Autodesk Fusion 360 part; units mm, degrees
(part 5 of 21)
  spline S66 degree 5 poles (-12.249, -28.4774) (-12.2425, -28.4716) (-12.2296, -28.4599) (-12.2103, -28.4423) (-12.1846, -28.4188) (-12.1527, -28.3894) (-12.1208, -28.3599) (-12.0891, -28.3303) (-12.0576, -28.3006) (-12.0261, -28.2709) (-11.9948, -28.241) (-11.9637, -28.2111) (-11.9326, -28.1811) (-11.9018, -28.151) (-11.871, -28.1208) (-11.8404, -28.0906) (-11.8099, -28.0602) (-11.7796, -28.0298) (-11.7494, -27.9993) (-11.7194, -27.9687) (-11.6895, -27.938) (-11.6597, -27.9072) (-11.6301, -27.8763) (-11.6007, -27.8454) (-11.5714, -27.8143) (-11.5422, -27.7832) (-11.5132, -27.752) (-11.4844, -27.7207) (-11.4557, -27.6893) (-11.4272, -27.6578) (-11.3988, -27.6262) (-11.3706, -27.5946) (-11.3426, -27.5628) (-11.3147, -27.5309) (-11.287, -27.499) (-11.2595, -27.467) (-11.2321, -27.4348) (-11.2049, -27.4026) (-11.1779, -27.3703) (-11.1511, -27.3379) (-11.1244, -27.3054) (-11.098, -27.2728) (-11.0717, -27.2401) (-11.0456, -27.2073) (-11.0197, -27.1743) (-10.994, -27.1413) (-10.9685, -27.1082) (-10.9432, -27.075) (-10.9181, -27.0417) (-10.8932, -27.0083) (-10.8686, -26.9747) (-10.8441, -26.9411) (-10.8199, -26.9073) (-10.7959, -26.8735) (-10.7721, -26.8395) (-10.752, -26.8103) (-10.7367, -26.7878) (-10.7261, -26.7721) (-10.7202, -26.7633) (-10.7188, -26.7613) knots -1 -1 -1 -1 -1 -1 -0.985714 -0.971429 -0.957143 -0.942857 -0.928571 -0.914286 -0.9 -0.885714 -0.871429 -0.857143 -0.842857 -0.828571 -0.814286 -0.8 -0.785714 -0.771429 -0.757143 -0.742857 -0.728571 -0.714286 -0.7 -0.685714 -0.671429 -0.657143 -0.642857 -0.628571 -0.614286 -0.6 -0.585714 -0.571429 -0.557143 -0.542857 -0.528571 -0.514286 -0.5 -0.485714 -0.471429 -0.457143 -0.442857 -0.428571 -0.414286 -0.4 -0.385714 -0.371429 -0.357143 -0.342857 -0.328571 -0.314286 -0.3 -0.285714 -0.271429 -0.257143 -0.242857 -0.228571 -0.224488 -0.224488 -0.224488 -0.224488 -0.224488 -0.224488
  spline S67 degree 3 poles (-10.599, -26.7241) (-10.6111, -26.7193) (-10.624, -26.7169) (-10.65, -26.7172) (-10.6629, -26.7199) (-10.6838, -26.7288) (-10.6921, -26.7338) (-10.7069, -26.7461) (-10.7135, -26.7533) (-10.7188, -26.7613) knots 0 0 0 0 0.003906 0.003906 0.007813 0.007813 0.010709 0.010709 0.013605 0.013605 0.013605 0.013605
  arc A64 (-10.599, -26.7241) -> (-10.0054, -26.952) centre (0, 0) ccw
  spline S68 degree 3 poles (-9.9412, -27.0598) (-9.9393, -27.047) (-9.94, -27.0338) (-9.9464, -27.0086) (-9.952, -26.9967) (-9.9655, -26.9785) (-9.9724, -26.9716) (-9.9878, -26.96) (-9.9963, -26.9553) (-10.0054, -26.952) knots 0 0 0 0 0.003906 0.003906 0.007813 0.007813 0.010709 0.010709 0.013605 0.013605 0.013605 0.013605
  spline S69 degree 5 poles (-9.9412, -27.0598) (-9.9415, -27.0622) (-9.943, -27.0727) (-9.9456, -27.0914) (-9.9493, -27.1184) (-9.9539, -27.1536) (-9.9589, -27.1948) (-9.9638, -27.236) (-9.9683, -27.2773) (-9.9727, -27.3186) (-9.9768, -27.3601) (-9.9807, -27.4015) (-9.9843, -27.4431) (-9.9878, -27.4847) (-9.991, -27.5264) (-9.994, -27.5681) (-9.9967, -27.6099) (-9.9993, -27.6517) (-10.0016, -27.6936) (-10.0038, -27.7355) (-10.0057, -27.7775) (-10.0075, -27.8196) (-10.0091, -27.8617) (-10.0104, -27.9038) (-10.0116, -27.946) (-10.0126, -27.9882) (-10.0133, -28.0305) (-10.0139, -28.0728) (-10.0144, -28.1152) (-10.0146, -28.1576) (-10.0146, -28.2) (-10.0145, -28.2425) (-10.0142, -28.285) (-10.0137, -28.3276) (-10.0131, -28.3702) (-10.0122, -28.4128) (-10.0112, -28.4555) (-10.01, -28.4982) (-10.0087, -28.541) (-10.0072, -28.5837) (-10.0055, -28.6265) (-10.0037, -28.6694) (-10.0016, -28.7123) (-9.9995, -28.7552) (-9.9971, -28.7981) (-9.9946, -28.8411) (-9.992, -28.8841) (-9.9892, -28.9271) (-9.9862, -28.9702) (-9.983, -29.0133) (-9.9798, -29.0564) (-9.9763, -29.0996) (-9.9727, -29.1427) (-9.9689, -29.1859) (-9.965, -29.2292) (-9.961, -29.2724) (-9.9576, -29.307) (-9.955, -29.333) (-9.9532, -29.3503) (-9.9524, -29.359) knots 0.224488 0.224488 0.224488 0.224488 0.224488 0.224488 0.228571 0.242857 0.257143 0.271429 0.285714 0.3 0.314286 0.328571 0.342857 0.357143 0.371429 0.385714 0.4 0.414286 0.428571 0.442857 0.457143 0.471429 0.485714 0.5 0.514286 0.528571 0.542857 0.557143 0.571429 0.585714 0.6 0.614286 0.628571 0.642857 0.657143 0.671429 0.685714 0.7 0.714286 0.728571 0.742857 0.757143 0.771429 0.785714 0.8 0.814286 0.828571 0.842857 0.857143 0.871429 0.885714 0.9 0.914286 0.928571 0.942857 0.957143 0.971429 0.985714 1 1 1 1 1 1
  arc A65 (-9.9524, -29.359) -> (-9.2052, -29.6018) centre (0, 0) ccw
  spline S70 degree 5 poles (-9.2052, -29.6018) (-9.1994, -29.5953) (-9.1877, -29.5823) (-9.1704, -29.5628) (-9.1473, -29.5368) (-9.1186, -29.5042) (-9.09, -29.4715) (-9.0616, -29.4388) (-9.0333, -29.406) (-9.0051, -29.3731) (-8.9771, -29.3401) (-8.9493, -29.3071) (-8.9215, -29.274) (-8.894, -29.2409) (-8.8665, -29.2076) (-8.8393, -29.1743) (-8.8121, -29.141) (-8.7851, -29.1075) (-8.7583, -29.074) (-8.7316, -29.0405) (-8.7051, -29.0068) (-8.6787, -28.9731) (-8.6525, -28.9393) (-8.6265, -28.9054) (-8.6006, -28.8715) (-8.5748, -28.8375) (-8.5493, -28.8034) (-8.5239, -28.7693) (-8.4986, -28.735) (-8.4735, -28.7007) (-8.4486, -28.6664) (-8.4239, -28.6319) (-8.3993, -28.5974) (-8.3749, -28.5628) (-8.3507, -28.5282) (-8.3267, -28.4934) (-8.3028, -28.4586) (-8.2792, -28.4237) (-8.2557, -28.3888) (-8.2324, -28.3537) (-8.2093, -28.3186) (-8.1864, -28.2834) (-8.1637, -28.2481) (-8.1412, -28.2128) (-8.1188, -28.1774) (-8.0967, -28.1418) (-8.0748, -28.1062) (-8.0531, -28.0706) (-8.0317, -28.0348) (-8.0104, -27.999) (-7.9894, -27.963) (-7.9686, -27.927) (-7.9481, -27.8909) (-7.9277, -27.8547) (-7.9076, -27.8185) (-7.8907, -27.7873) (-7.8778, -27.7633) (-7.8689, -27.7466) (-7.8639, -27.7372) (-7.8628, -27.7352) knots -1 -1 -1 -1 -1 -1 -0.985714 -0.971429 -0.957143 -0.942857 -0.928571 -0.914286 -0.9 -0.885714 -0.871429 -0.857143 -0.842857 -0.828571 -0.814286 -0.8 -0.785714 -0.771429 -0.757143 -0.742857 -0.728571 -0.714286 -0.7 -0.685714 -0.671429 -0.657143 -0.642857 -0.628571 -0.614286 -0.6 -0.585714 -0.571429 -0.557143 -0.542857 -0.528571 -0.514286 -0.5 -0.485714 -0.471429 -0.457143 -0.442857 -0.428571 -0.414286 -0.4 -0.385714 -0.371429 -0.357143 -0.342857 -0.328571 -0.314286 -0.3 -0.285714 -0.271429 -0.257143 -0.242857 -0.228571 -0.224488 -0.224488 -0.224488 -0.224488 -0.224488 -0.224488
  spline S71 degree 3 poles (-7.7475, -27.6856) (-7.76, -27.6821) (-7.7731, -27.6811) (-7.799, -27.6841) (-7.8115, -27.6881) (-7.8313, -27.6991) (-7.839, -27.705) (-7.8526, -27.7188) (-7.8583, -27.7266) (-7.8628, -27.7352) knots 0 0 0 0 0.003906 0.003906 0.007813 0.007813 0.010709 0.010709 0.013605 0.013605 0.013605 0.013605
  arc A66 (-7.7475, -27.6856) -> (-7.1333, -27.8502) centre (0, 0) ccw
  spline S72 degree 3 poles (-7.0582, -27.9507) (-7.0577, -27.9377) (-7.0598, -27.9248) (-7.0688, -27.9003) (-7.0756, -27.8891) (-7.0909, -27.8724) (-7.0984, -27.8662) (-7.115, -27.8563) (-7.124, -27.8526) (-7.1333, -27.8502) knots 0 0 0 0 0.003906 0.003906 0.007813 0.007813 0.010709 0.010709 0.013605 0.013605 0.013605 0.013605
  spline S73 degree 5 poles (-7.0582, -27.9507) (-7.0583, -27.9531) (-7.0587, -27.9637) (-7.0593, -27.9826) (-7.0601, -28.0098) (-7.061, -28.0453) (-7.0618, -28.0868) (-7.0622, -28.1283) (-7.0625, -28.1698) (-7.0625, -28.2114) (-7.0622, -28.253) (-7.0618, -28.2947) (-7.0611, -28.3364) (-7.0601, -28.3781) (-7.059, -28.4199) (-7.0576, -28.4617) (-7.0559, -28.5036) (-7.0541, -28.5454) (-7.0521, -28.5873) (-7.0498, -28.6293) (-7.0474, -28.6712) (-7.0447, -28.7132) (-7.0419, -28.7553) (-7.0388, -28.7973) (-7.0356, -28.8394) (-7.0321, -28.8815) (-7.0285, -28.9236) (-7.0247, -28.9658) (-7.0207, -29.0079) (-7.0165, -29.0501) (-7.0121, -29.0923) (-7.0075, -29.1346) (-7.0027, -29.1768) (-6.9978, -29.2191) (-6.9927, -29.2614) (-6.9874, -29.3037) (-6.982, -29.3461) (-6.9763, -29.3884) (-6.9705, -29.4308) (-6.9646, -29.4732) (-6.9584, -29.5156) (-6.9521, -29.558) (-6.9456, -29.6004) (-6.939, -29.6429) (-6.9321, -29.6854) (-6.9252, -29.7278) (-6.918, -29.7703) (-6.9107, -29.8128) (-6.9033, -29.8553) (-6.8956, -29.8979) (-6.8879, -29.9404) (-6.8799, -29.983) (-6.8718, -30.0255) (-6.8636, -30.0681) (-6.8552, -30.1107) (-6.8466, -30.1533) (-6.8396, -30.1873) (-6.8343, -30.2129) (-6.8308, -30.2299) (-6.829, -30.2385) knots 0.224488 0.224488 0.224488 0.224488 0.224488 0.224488 0.228571 0.242857 0.257143 0.271429 0.285714 0.3 0.314286 0.328571 0.342857 0.357143 0.371429 0.385714 0.4 0.414286 0.428571 0.442857 0.457143 0.471429 0.485714 0.5 0.514286 0.528571 0.542857 0.557143 0.571429 0.585714 0.6 0.614286 0.628571 0.642857 0.657143 0.671429 0.685714 0.7 0.714286 0.728571 0.742857 0.757143 0.771429 0.785714 0.8 0.814286 0.828571 0.842857 0.857143 0.871429 0.885714 0.9 0.914286 0.928571 0.942857 0.957143 0.971429 0.985714 1 1 1 1 1 1
  arc A67 (-6.829, -30.2385) -> (-6.0605, -30.4018) centre (0, 0) ccw
  spline S74 degree 5 poles (-6.0605, -30.4018) (-6.0554, -30.3948) (-6.0452, -30.3806) (-6.03, -30.3594) (-6.0097, -30.3311) (-5.9846, -30.2957) (-5.9596, -30.2602) (-5.9348, -30.2247) (-5.91, -30.1891) (-5.8855, -30.1535) (-5.8611, -30.1178) (-5.8368, -30.082) (-5.8127, -30.0462) (-5.7887, -30.0104) (-5.7649, -29.9744) (-5.7413, -29.9385) (-5.7178, -29.9025) (-5.6945, -29.8664) (-5.6713, -29.8303) (-5.6483, -29.7941) (-5.6254, -29.7578) (-5.6027, -29.7215) (-5.5802, -29.6852) (-5.5578, -29.6488) (-5.5356, -29.6123) (-5.5135, -29.5758) (-5.4917, -29.5393) (-5.47, -29.5026) (-5.4484, -29.466) (-5.4271, -29.4292) (-5.4059, -29.3925) (-5.3849, -29.3556) (-5.3641, -29.3187) (-5.3434, -29.2818) (-5.323, -29.2448) (-5.3027, -29.2077) (-5.2826, -29.1706) (-5.2627, -29.1334) (-5.243, -29.0962) (-5.2235, -29.0589) (-5.2042, -29.0216) (-5.1851, -28.9842) (-5.1662, -28.9467) (-5.1475, -28.9092) (-5.129, -28.8716) (-5.1107, -28.834) (-5.0927, -28.7963) (-5.0749, -28.7586) (-5.0572, -28.7208) (-5.0399, -28.6829) (-5.0227, -28.645) (-5.0058, -28.607) (-4.9891, -28.5689) (-4.9727, -28.5308) (-4.9565, -28.4926) (-4.9429, -28.4599) (-4.9326, -28.4347) (-4.9255, -28.4172) (-4.9215, -28.4073) (-4.9206, -28.4051) knots -1 -1 -1 -1 -1 -1 -0.985714 -0.971429 -0.957143 -0.942857 -0.928571 -0.914286 -0.9 -0.885714 -0.871429 -0.857143 -0.842857 -0.828571 -0.814286 -0.8 -0.785714 -0.771429 -0.757143 -0.742857 -0.728571 -0.714286 -0.7 -0.685714 -0.671429 -0.657143 -0.642857 -0.628571 -0.614286 -0.6 -0.585714 -0.571429 -0.557143 -0.542857 -0.528571 -0.514286 -0.5 -0.485714 -0.471429 -0.457143 -0.442857 -0.428571 -0.414286 -0.4 -0.385714 -0.371429 -0.357143 -0.342857 -0.328571 -0.314286 -0.3 -0.285714 -0.271429 -0.257143 -0.242857 -0.228571 -0.224488 -0.224488 -0.224488 -0.224488 -0.224488 -0.224488
  spline S75 degree 3 poles (-4.8111, -28.3438) (-4.8239, -28.3416) (-4.8371, -28.342) (-4.8625, -28.3477) (-4.8745, -28.353) (-4.8931, -28.366) (-4.9001, -28.3726) (-4.9121, -28.3878) (-4.917, -28.3961) (-4.9206, -28.4051) knots 0 0 0 0 0.003906 0.003906 0.007813 0.007813 0.010709 0.010709 0.013605 0.013605 0.013605 0.013605
  arc A68 (-4.8111, -28.3438) -> (-4.1831, -28.4432) centre (0, 0) ccw
  spline S76 degree 3 poles (-4.0979, -28.5354) (-4.0988, -28.5224) (-4.1022, -28.5097) (-4.1137, -28.4864) (-4.1216, -28.4759) (-4.1386, -28.4609) (-4.1467, -28.4556) (-4.1642, -28.4474) (-4.1735, -28.4447) (-4.1831, -28.4432) knots 0 0 0 0 0.003906 0.003906 0.007813 0.007813 0.010709 0.010709 0.013605 0.013605 0.013605 0.013605
  spline S77 degree 5 poles (-4.0979, -28.5354) (-4.0977, -28.5378) (-4.097, -28.5484) (-4.0957, -28.5672) (-4.0936, -28.5944) (-4.0908, -28.6298) (-4.0872, -28.6711) (-4.0833, -28.7124) (-4.0792, -28.7537) (-4.0749, -28.7951) (-4.0703, -28.8365) (-4.0655, -28.8778) (-4.0604, -28.9192) (-4.0551, -28.9607) (-4.0496, -29.0021) (-4.0438, -29.0435) (-4.0379, -29.085) (-4.0317, -29.1264) (-4.0253, -29.1679) (-4.0186, -29.2094) (-4.0118, -29.2508) (-4.0048, -29.2923) (-3.9976, -29.3338) (-3.9901, -29.3753) (-3.9825, -29.4168) (-3.9747, -29.4583) (-3.9667, -29.4998) (-3.9584, -29.5414) (-3.95, -29.5829) (-3.9415, -29.6244) (-3.9327, -29.6659) (-3.9237, -29.7075) (-3.9146, -29.749) (-3.9053, -29.7905) (-3.8958, -29.8321) (-3.8861, -29.8736) (-3.8762, -29.9151) (-3.8662, -29.9567) (-3.856, -29.9982) (-3.8456, -30.0397) (-3.8351, -30.0812) (-3.8244, -30.1228) (-3.8135, -30.1643) (-3.8024, -30.2058) (-3.7912, -30.2473) (-3.7798, -30.2889) (-3.7683, -30.3304) (-3.7566, -30.3719) (-3.7447, -30.4134) (-3.7327, -30.4549) (-3.7205, -30.4964) (-3.7082, -30.5379) (-3.6957, -30.5793) (-3.683, -30.6208) (-3.6702, -30.6623) (-3.6572, -30.7037) (-3.6467, -30.7369) (-3.6388, -30.7618) (-3.6335, -30.7784) (-3.6308, -30.7866) knots 0.224488 0.224488 0.224488 0.224488 0.224488 0.224488 0.228571 0.242857 0.257143 0.271429 0.285714 0.3 0.314286 0.328571 0.342857 0.357143 0.371429 0.385714 0.4 0.414286 0.428571 0.442857 0.457143 0.471429 0.485714 0.5 0.514286 0.528571 0.542857 0.557143 0.571429 0.585714 0.6 0.614286 0.628571 0.642857 0.657143 0.671429 0.685714 0.7 0.714286 0.728571 0.742857 0.757143 0.771429 0.785714 0.8 0.814286 0.828571 0.842857 0.857143 0.871429 0.885714 0.9 0.914286 0.928571 0.942857 0.957143 0.971429 0.985714 1 1 1 1 1 1
  arc A69 (-3.6308, -30.7866) -> (-2.8495, -30.8688) centre (0, 0) ccw
  spline S78 degree 5 poles (-2.8495, -30.8688) (-2.8451, -30.8612) (-2.8365, -30.8461) (-2.8235, -30.8234) (-2.8064, -30.7932) (-2.7851, -30.7553) (-2.7639, -30.7174) (-2.7429, -30.6795) (-2.722, -30.6415) (-2.7013, -30.6035) (-2.6808, -30.5654) (-2.6604, -30.5273) (-2.6402, -30.4892) (-2.6201, -30.451) (-2.6002, -30.4128) (-2.5804, -30.3746) (-2.5608, -30.3363) (-2.5414, -30.298) (-2.5221, -30.2596) (-2.503, -30.2213) (-2.484, -30.1828) (-2.4653, -30.1444) (-2.4466, -30.1059) (-2.4282, -30.0673) (-2.4099, -30.0287) (-2.3918, -29.9901) (-2.3739, -29.9515) (-2.3561, -29.9128) (-2.3386, -29.8741) (-2.3212, -29.8353) (-2.3039, -29.7965) (-2.2869, -29.7577) (-2.2701, -29.7188) (-2.2534, -29.6799) (-2.2369, -29.641) (-2.2206, -29.602) (-2.2045, -29.563) (-2.1886, -29.5239) (-2.1729, -29.4849) (-2.1574, -29.4457) (-2.1421, -29.4066) (-2.127, -29.3674) (-2.1122, -29.3282) (-2.0975, -29.2889) (-2.083, -29.2496) (-2.0688, -29.2103) (-2.0548, -29.1709) (-2.041, -29.1315) (-2.0274, -29.0921) (-2.0141, -29.0526) (-2.001, -29.0131) (-1.9881, -28.9735) (-1.9755, -28.9339) (-1.9632, -28.8943) (-1.9511, -28.8546) (-1.9409, -28.8206) (-1.9333, -28.7945) (-1.9281, -28.7763) (-1.9252, -28.7661) (-1.9245, -28.7638) knots -1 -1 -1 -1 -1 -1 -0.985714 -0.971429 -0.957143 -0.942857 -0.928571 -0.914286 -0.9 -0.885714 -0.871429 -0.857143 -0.842857 -0.828571 -0.814286 -0.8 -0.785714 -0.771429 -0.757143 -0.742857 -0.728571 -0.714286 -0.7 -0.685714 -0.671429 -0.657143 -0.642857 -0.628571 -0.614286 -0.6 -0.585714 -0.571429 -0.557143 -0.542857 -0.528571 -0.514286 -0.5 -0.485714 -0.471429 -0.457143 -0.442857 -0.428571 -0.414286 -0.4 -0.385714 -0.371429 -0.357143 -0.342857 -0.328571 -0.314286 -0.3 -0.285714 -0.271429 -0.257143 -0.242857 -0.228571 -0.224488 -0.224488 -0.224488 -0.224488 -0.224488 -0.224488
  spline S79 degree 3 poles (-1.822, -28.6914) (-1.835, -28.6906) (-1.848, -28.6923) (-1.8727, -28.7006) (-1.8841, -28.7072) (-1.9012, -28.7221) (-1.9075, -28.7294) (-1.9179, -28.7457) (-1.9219, -28.7546) (-1.9245, -28.7638) knots 0 0 0 0 0.003906 0.003906 0.007813 0.007813 0.010709 0.010709 0.013605 0.013605 0.013605 0.013605
  arc A70 (-1.822, -28.6914) -> (-1.1871, -28.7247) centre (0, 0) ccw
  spline S80 degree 3 poles (-1.0927, -28.8074) (-1.0949, -28.7946) (-1.0996, -28.7823) (-1.1135, -28.7603) (-1.1225, -28.7507) (-1.141, -28.7376) (-1.1496, -28.7331) (-1.1679, -28.7269) (-1.1774, -28.7251) (-1.1871, -28.7247) knots 0 0 0 0 0.003906 0.003906 0.007813 0.007813 0.010709 0.010709 0.013605 0.013605 0.013605 0.013605
  spline S81 degree 5 poles (-1.0927, -28.8074) (-1.0923, -28.8098) (-1.0904, -28.8202) (-1.0871, -28.8389) (-1.0823, -28.8656) (-1.0758, -28.9005) (-1.0679, -28.9412) (-1.0597, -28.9819) (-1.0513, -29.0226) (-1.0427, -29.0633) (-1.0338, -29.104) (-1.0247, -29.1446) (-1.0153, -29.1853) (-1.0057, -29.2259) (-0.9959, -29.2665) (-0.9858, -29.3071) (-0.9755, -29.3477) (-0.965, -29.3883) (-0.9543, -29.4289) (-0.9434, -29.4694) (-0.9323, -29.5099) (-0.921, -29.5505) (-0.9094, -29.591) (-0.8977, -29.6315) (-0.8858, -29.672) (-0.8737, -29.7124) (-0.8614, -29.7529) (-0.8488, -29.7933) (-0.8361, -29.8337) (-0.8233, -29.8741) (-0.8102, -29.9145) (-0.7969, -29.9549) (-0.7835, -29.9952) (-0.7699, -30.0355) (-0.7561, -30.0759) (-0.7421, -30.1161) (-0.728, -30.1564) (-0.7137, -30.1967) (-0.6992, -30.2369) (-0.6845, -30.2771) (-0.6697, -30.3173) (-0.6547, -30.3575) (-0.6396, -30.3977) (-0.6242, -30.4378) (-0.6087, -30.4779) (-0.5931, -30.518) (-0.5773, -30.5581) (-0.5613, -30.5982) (-0.5451, -30.6382) (-0.5288, -30.6782) (-0.5124, -30.7182) (-0.4958, -30.7582) (-0.479, -30.7981) (-0.4621, -30.838) (-0.445, -30.8779) (-0.4278, -30.9178) (-0.4139, -30.9497) (-0.4034, -30.9736) (-0.3963, -30.9895) (-0.3928, -30.9975) knots 0.224488 0.224488 0.224488 0.224488 0.224488 0.224488 0.228571 0.242857 0.257143 0.271429 0.285714 0.3 0.314286 0.328571 0.342857 0.357143 0.371429 0.385714 0.4 0.414286 0.428571 0.442857 0.457143 0.471429 0.485714 0.5 0.514286 0.528571 0.542857 0.557143 0.571429 0.585714 0.6 0.614286 0.628571 0.642857 0.657143 0.671429 0.685714 0.7 0.714286 0.728571 0.742857 0.757143 0.771429 0.785714 0.8 0.814286 0.828571 0.842857 0.857143 0.871429 0.885714 0.9 0.914286 0.928571 0.942857 0.957143 0.971429 0.985714 1 1 1 1 1 1
  arc A71 (-0.3928, -30.9975) -> (0.3928, -30.9975) centre (0, 0) ccw
  spline S82 degree 5 poles (0.3928, -30.9975) (0.3963, -30.9895) (0.4034, -30.9736) (0.4139, -30.9497) (0.4278, -30.9178) (0.445, -30.8779) (0.4621, -30.838) (0.479, -30.7981) (0.4958, -30.7582) (0.5124, -30.7182) (0.5288, -30.6782) (0.5451, -30.6382) (0.5613, -30.5982) (0.5773, -30.5581) (0.5931, -30.518) (0.6087, -30.4779) (0.6242, -30.4378) (0.6396, -30.3977) (0.6547, -30.3575) (0.6697, -30.3173) (0.6845, -30.2771) (0.6992, -30.2369) (0.7137, -30.1967) (0.728, -30.1564) (0.7421, -30.1161) (0.7561, -30.0759) (0.7699, -30.0355) (0.7835, -29.9952) (0.7969, -29.9549) (0.8102, -29.9145) (0.8233, -29.8741) (0.8361, -29.8337) (0.8488, -29.7933) (0.8614, -29.7529) (0.8737, -29.7124) (0.8858, -29.672) (0.8977, -29.6315) (0.9094, -29.591) (0.921, -29.5505) (0.9323, -29.5099) (0.9434, -29.4694) (0.9543, -29.4289) (0.965, -29.3883) (0.9755, -29.3477) (0.9858, -29.3071) (0.9959, -29.2665) (1.0057, -29.2259) (1.0153, -29.1853) (1.0247, -29.1446) (1.0338, -29.104) (1.0427, -29.0633) (1.0513, -29.0226) (1.0597, -28.9819) (1.0679, -28.9412) (1.0758, -28.9005) (1.0823, -28.8656) (1.0871, -28.8389) (1.0904, -28.8202) (1.0923, -28.8098) (1.0927, -28.8074) knots -1 -1 -1 -1 -1 -1 -0.985714 -0.971429 -0.957143 -0.942857 -0.928571 -0.914286 -0.9 -0.885714 -0.871429 -0.857143 -0.842857 -0.828571 -0.814286 -0.8 -0.785714 -0.771429 -0.757143 -0.742857 -0.728571 -0.714286 -0.7 -0.685714 -0.671429 -0.657143 -0.642857 -0.628571 -0.614286 -0.6 -0.585714 -0.571429 -0.557143 -0.542857 -0.528571 -0.514286 -0.5 -0.485714 -0.471429 -0.457143 -0.442857 -0.428571 -0.414286 -0.4 -0.385714 -0.371429 -0.357143 -0.342857 -0.328571 -0.314286 -0.3 -0.285714 -0.271429 -0.257143 -0.242857 -0.228571 -0.224488 -0.224488 -0.224488 -0.224488 -0.224488 -0.224488
  spline S83 degree 3 poles (1.1871, -28.7247) (1.174, -28.7252) (1.1613, -28.7283) (1.1376, -28.7392) (1.1269, -28.7469) (1.1115, -28.7634) (1.1059, -28.7714) (1.0973, -28.7887) (1.0943, -28.7979) (1.0927, -28.8074) knots 0 0 0 0 0.003906 0.003906 0.007813 0.007813 0.010709 0.010709 0.013605 0.013605 0.013605 0.013605
  arc A72 (1.1871, -28.7247) -> (1.822, -28.6914) centre (0, 0) ccw
  spline S84 degree 3 poles (1.9245, -28.7638) (1.921, -28.7513) (1.915, -28.7396) (1.8989, -28.7191) (1.8889, -28.7106) (1.8692, -28.6994) (1.8601, -28.6959) (1.8413, -28.6916) (1.8316, -28.6908) (1.822, -28.6914) knots 0 0 0 0 0.003906 0.003906 0.007813 0.007813 0.010709 0.010709 0.013605 0.013605 0.013605 0.013605
  spline S85 degree 5 poles (1.9245, -28.7638) (1.9252, -28.7661) (1.9281, -28.7763) (1.9333, -28.7945) (1.9409, -28.8206) (1.9511, -28.8546) (1.9632, -28.8943) (1.9755, -28.9339) (1.9881, -28.9735) (2.001, -29.0131) (2.0141, -29.0526) (2.0274, -29.0921) (2.041, -29.1315) (2.0548, -29.1709) (2.0688, -29.2103) (2.083, -29.2496) (2.0975, -29.2889) (2.1122, -29.3282) (2.127, -29.3674) (2.1421, -29.4066) (2.1574, -29.4457) (2.1729, -29.4849) (2.1886, -29.5239) (2.2045, -29.563) (2.2206, -29.602) (2.2369, -29.641) (2.2534, -29.6799) (2.2701, -29.7188) (2.2869, -29.7577) (2.3039, -29.7965) (2.3212, -29.8353) (2.3386, -29.8741) (2.3561, -29.9128) (2.3739, -29.9515) (2.3918, -29.9901) (2.4099, -30.0287) (2.4282, -30.0673) (2.4466, -30.1059) (2.4653, -30.1444) (2.484, -30.1828) (2.503, -30.2213) (2.5221, -30.2596) (2.5414, -30.298) (2.5608, -30.3363) (2.5804, -30.3746) (2.6002, -30.4128) (2.6201, -30.451) (2.6402, -30.4892) (2.6604, -30.5273) (2.6808, -30.5654) (2.7013, -30.6035) (2.722, -30.6415) (2.7429, -30.6795) (2.7639, -30.7174) (2.7851, -30.7553) (2.8064, -30.7932) (2.8235, -30.8234) (2.8365, -30.8461) (2.8451, -30.8612) (2.8495, -30.8688) knots 0.224488 0.224488 0.224488 0.224488 0.224488 0.224488 0.228571 0.242857 0.257143 0.271429 0.285714 0.3 0.314286 0.328571 0.342857 0.357143 0.371429 0.385714 0.4 0.414286 0.428571 0.442857 0.457143 0.471429 0.485714 0.5 0.514286 0.528571 0.542857 0.557143 0.571429 0.585714 0.6 0.614286 0.628571 0.642857 0.657143 0.671429 0.685714 0.7 0.714286 0.728571 0.742857 0.757143 0.771429 0.785714 0.8 0.814286 0.828571 0.842857 0.857143 0.871429 0.885714 0.9 0.914286 0.928571 0.942857 0.957143 0.971429 0.985714 1 1 1 1 1 1
  arc A73 (2.8495, -30.8688) -> (3.6308, -30.7866) centre (0, 0) ccw
  spline S86 degree 5 poles (3.6308, -30.7866) (3.6335, -30.7784) (3.6388, -30.7618) (3.6467, -30.7369) (3.6572, -30.7037) (3.6702, -30.6623) (3.683, -30.6208) (3.6957, -30.5793) (3.7082, -30.5379) (3.7205, -30.4964) (3.7327, -30.4549) (3.7447, -30.4134) (3.7566, -30.3719) (3.7683, -30.3304) (3.7798, -30.2889) (3.7912, -30.2473) (3.8024, -30.2058) (3.8135, -30.1643) (3.8244, -30.1228) (3.8351, -30.0812) (3.8456, -30.0397) (3.856, -29.9982) (3.8662, -29.9567) (3.8762, -29.9151) (3.8861, -29.8736) (3.8958, -29.8321) (3.9053, -29.7905) (3.9146, -29.749) (3.9237, -29.7075) (3.9327, -29.6659) (3.9415, -29.6244) (3.95, -29.5829) (3.9584, -29.5414) (3.9667, -29.4998) (3.9747, -29.4583) (3.9825, -29.4168) (3.9901, -29.3753) (3.9976, -29.3338) (4.0048, -29.2923) (4.0118, -29.2508) (4.0186, -29.2094) (4.0253, -29.1679) (4.0317, -29.1264) (4.0379, -29.085) (4.0438, -29.0435) (4.0496, -29.0021) (4.0551, -28.9607) (4.0604, -28.9192) (4.0655, -28.8778) (4.0703, -28.8365) (4.0749, -28.7951) (4.0792, -28.7537) (4.0833, -28.7124) (4.0872, -28.6711) (4.0908, -28.6298) (4.0936, -28.5944) (4.0957, -28.5672) (4.097, -28.5484) (4.0977, -28.5378) (4.0979, -28.5354) knots -1 -1 -1 -1 -1 -1 -0.985714 -0.971429 -0.957143 -0.942857 -0.928571 -0.914286 -0.9 -0.885714 -0.871429 -0.857143 -0.842857 -0.828571 -0.814286 -0.8 -0.785714 -0.771429 -0.757143 -0.742857 -0.728571 -0.714286 -0.7 -0.685714 -0.671429 -0.657143 -0.642857 -0.628571 -0.614286 -0.6 -0.585714 -0.571429 -0.557143 -0.542857 -0.528571 -0.514286 -0.5 -0.485714 -0.471429 -0.457143 -0.442857 -0.428571 -0.414286 -0.4 -0.385714 -0.371429 -0.357143 -0.342857 -0.328571 -0.314286 -0.3 -0.285714 -0.271429 -0.257143 -0.242857 -0.228571 -0.224488 -0.224488 -0.224488 -0.224488 -0.224488 -0.224488
  spline S87 degree 3 poles (4.1831, -28.4432) (4.1702, -28.4451) (4.1578, -28.4495) (4.1354, -28.4628) (4.1256, -28.4716) (4.112, -28.4897) (4.1073, -28.4982) (4.1006, -28.5163) (4.0985, -28.5258) (4.0979, -28.5354) knots 0 0 0 0 0.003906 0.003906 0.007813 0.007813 0.010709 0.010709 0.013605 0.013605 0.013605 0.013605
  arc A74 (4.1831, -28.4432) -> (4.8111, -28.3438) centre (0, 0) ccw
  spline S88 degree 3 poles (4.9206, -28.4051) (4.9158, -28.393) (4.9086, -28.382) (4.8904, -28.3633) (4.8796, -28.3559) (4.8588, -28.3468) (4.8495, -28.3443) (4.8303, -28.3419) (4.8206, -28.3422) (4.8111, -28.3438) knots 0 0 0 0 0.003906 0.003906 0.007813 0.007813 0.010709 0.010709 0.013605 0.013605 0.013605 0.013605
  spline S89 degree 5 poles (4.9206, -28.4051) (4.9215, -28.4073) (4.9255, -28.4172) (4.9326, -28.4347) (4.9429, -28.4599) (4.9565, -28.4926) (4.9727, -28.5308) (4.9891, -28.5689) (5.0058, -28.607) (5.0227, -28.645) (5.0399, -28.6829) (5.0572, -28.7208) (5.0749, -28.7586) (5.0927, -28.7963) (5.1107, -28.834) (5.129, -28.8716) (5.1475, -28.9092) (5.1662, -28.9467) (5.1851, -28.9842) (5.2042, -29.0216) (5.2235, -29.0589) (5.243, -29.0962) (5.2627, -29.1334) (5.2826, -29.1706) (5.3027, -29.2077) (5.323, -29.2448) (5.3434, -29.2818) (5.3641, -29.3187) (5.3849, -29.3556) (5.4059, -29.3925) (5.4271, -29.4292) (5.4484, -29.466) (5.47, -29.5026) (5.4917, -29.5393) (5.5135, -29.5758) (5.5356, -29.6123) (5.5578, -29.6488) (5.5802, -29.6852) (5.6027, -29.7215) (5.6254, -29.7578) (5.6483, -29.7941) (5.6713, -29.8303) (5.6945, -29.8664) (5.7178, -29.9025) (5.7413, -29.9385) (5.7649, -29.9744) (5.7887, -30.0104) (5.8127, -30.0462) (5.8368, -30.082) (5.8611, -30.1178) (5.8855, -30.1535) (5.91, -30.1891) (5.9348, -30.2247) (5.9596, -30.2602) (5.9846, -30.2957) (6.0097, -30.3311) (6.03, -30.3594) (6.0452, -30.3806) (6.0554, -30.3948) (6.0605, -30.4018) knots 0.224488 0.224488 0.224488 0.224488 0.224488 0.224488 0.228571 0.242857 0.257143 0.271429 0.285714 0.3 0.314286 0.328571 0.342857 0.357143 0.371429 0.385714 0.4 0.414286 0.428571 0.442857 0.457143 0.471429 0.485714 0.5 0.514286 0.528571 0.542857 0.557143 0.571429 0.585714 0.6 0.614286 0.628571 0.642857 0.657143 0.671429 0.685714 0.7 0.714286 0.728571 0.742857 0.757143 0.771429 0.785714 0.8 0.814286 0.828571 0.842857 0.857143 0.871429 0.885714 0.9 0.914286 0.928571 0.942857 0.957143 0.971429 0.985714 1 1 1 1 1 1
  arc A75 (6.0605, -30.4018) -> (6.829, -30.2385) centre (0, 0) ccw
  spline S90 degree 5 poles (6.829, -30.2385) (6.8308, -30.2299) (6.8343, -30.2129) (6.8396, -30.1873) (6.8466, -30.1533) (6.8552, -30.1107) (6.8636, -30.0681) (6.8718, -30.0255) (6.8799, -29.983) (6.8879, -29.9404) (6.8956, -29.8979) (6.9033, -29.8553) (6.9107, -29.8128) (6.918, -29.7703) (6.9252, -29.7278) (6.9321, -29.6854) (6.939, -29.6429) (6.9456, -29.6004) (6.9521, -29.558) (6.9584, -29.5156) (6.9646, -29.4732) (6.9705, -29.4308) (6.9763, -29.3884) (6.982, -29.3461) (6.9874, -29.3037) (6.9927, -29.2614) (6.9978, -29.2191) (7.0027, -29.1768) (7.0075, -29.1346) (7.0121, -29.0923) (7.0165, -29.0501) (7.0207, -29.0079) (7.0247, -28.9658) (7.0285, -28.9236) (7.0321, -28.8815) (7.0356, -28.8394) (7.0388, -28.7973) (7.0419, -28.7553) (7.0447, -28.7132) (7.0474, -28.6712) (7.0498, -28.6293) (7.0521, -28.5873) (7.0541, -28.5454) (7.0559, -28.5036) (7.0576, -28.4617) (7.059, -28.4199) (7.0601, -28.3781) (7.0611, -28.3364) (7.0618, -28.2947) (7.0622, -28.253) (7.0625, -28.2114) (7.0625, -28.1698) (7.0622, -28.1283) (7.0618, -28.0868) (7.061, -28.0453) (7.0601, -28.0098) (7.0593, -27.9826) (7.0587, -27.9637) (7.0583, -27.9531) (7.0582, -27.9507) knots -1 -1 -1 -1 -1 -1 -0.985714 -0.971429 -0.957143 -0.942857 -0.928571 -0.914286 -0.9 -0.885714 -0.871429 -0.857143 -0.842857 -0.828571 -0.814286 -0.8 -0.785714 -0.771429 -0.757143 -0.742857 -0.728571 -0.714286 -0.7 -0.685714 -0.671429 -0.657143 -0.642857 -0.628571 -0.614286 -0.6 -0.585714 -0.571429 -0.557143 -0.542857 -0.528571 -0.514286 -0.5 -0.485714 -0.471429 -0.457143 -0.442857 -0.428571 -0.414286 -0.4 -0.385714 -0.371429 -0.357143 -0.342857 -0.328571 -0.314286 -0.3 -0.285714 -0.271429 -0.257143 -0.242857 -0.228571 -0.224488 -0.224488 -0.224488 -0.224488 -0.224488 -0.224488
  spline S91 degree 3 poles (7.1333, -27.8502) (7.1207, -27.8534) (7.1088, -27.8591) (7.0879, -27.8746) (7.0791, -27.8844) (7.0674, -27.9038) (7.0637, -27.9128) (7.0589, -27.9315) (7.0578, -27.9411) (7.0582, -27.9507) knots 0 0 0 0 0.003906 0.003906 0.007813 0.007813 0.010709 0.010709 0.013605 0.013605 0.013605 0.013605
  arc A76 (7.1333, -27.8502) -> (7.7475, -27.6856) centre (0, 0) ccw
  spline S92 degree 3 poles (7.8628, -27.7352) (7.8567, -27.7236) (7.8484, -27.7134) (7.8284, -27.6968) (7.8169, -27.6905) (7.7953, -27.6836) (7.7857, -27.6821) (7.7664, -27.6818) (7.7568, -27.683) (7.7475, -27.6856) knots 0 0 0 0 0.003906 0.003906 0.007813 0.007813 0.010709 0.010709 0.013605 0.013605 0.013605 0.013605
  spline S93 degree 5 poles (7.8628, -27.7352) (7.8639, -27.7372) (7.8689, -27.7466) (7.8778, -27.7633) (7.8907, -27.7873) (7.9076, -27.8185) (7.9277, -27.8547) (7.9481, -27.8909) (7.9686, -27.927) (7.9894, -27.963) (8.0104, -27.999) (8.0317, -28.0348) (8.0531, -28.0706) (8.0748, -28.1062) (8.0967, -28.1418) (8.1188, -28.1774) (8.1412, -28.2128) (8.1637, -28.2481) (8.1864, -28.2834) (8.2093, -28.3186) (8.2324, -28.3537) (8.2557, -28.3888) (8.2792, -28.4237) (8.3028, -28.4586) (8.3267, -28.4934) (8.3507, -28.5282) (8.3749, -28.5628) (8.3993, -28.5974) (8.4239, -28.6319) (8.4486, -28.6664) (8.4735, -28.7007) (8.4986, -28.735) (8.5239, -28.7693) (8.5493, -28.8034) (8.5748, -28.8375) (8.6006, -28.8715) (8.6265, -28.9054) (8.6525, -28.9393) (8.6787, -28.9731) (8.7051, -29.0068) (8.7316, -29.0405) (8.7583, -29.074) (8.7851, -29.1075) (8.8121, -29.141) (8.8393, -29.1743) (8.8665, -29.2076) (8.894, -29.2409) (8.9215, -29.274) (8.9493, -29.3071) (8.9771, -29.3401) (9.0051, -29.3731) (9.0333, -29.406) (9.0616, -29.4388) (9.09, -29.4715) (9.1186, -29.5042) (9.1473, -29.5368) (9.1704, -29.5628) (9.1877, -29.5823) (9.1994, -29.5953) (9.2052, -29.6018) knots 0.224488 0.224488 0.224488 0.224488 0.224488 0.224488 0.228571 0.242857 0.257143 0.271429 0.285714 0.3 0.314286 0.328571 0.342857 0.357143 0.371429 0.385714 0.4 0.414286 0.428571 0.442857 0.457143 0.471429 0.485714 0.5 0.514286 0.528571 0.542857 0.557143 0.571429 0.585714 0.6 0.614286 0.628571 0.642857 0.657143 0.671429 0.685714 0.7 0.714286 0.728571 0.742857 0.757143 0.771429 0.785714 0.8 0.814286 0.828571 0.842857 0.857143 0.871429 0.885714 0.9 0.914286 0.928571 0.942857 0.957143 0.971429 0.985714 1 1 1 1 1 1
  arc A77 (9.2052, -29.6018) -> (9.9524, -29.359) centre (0, 0) ccw
  spline S94 degree 5 poles (9.9524, -29.359) (9.9532, -29.3503) (9.955, -29.333) (9.9576, -29.307) (9.961, -29.2724) (9.965, -29.2292) (9.9689, -29.1859) (9.9727, -29.1427) (9.9763, -29.0996) (9.9798, -29.0564) (9.983, -29.0133) (9.9862, -28.9702) (9.9892, -28.9271) (9.992, -28.8841) (9.9946, -28.8411) (9.9971, -28.7981) (9.9995, -28.7552) (10.0016, -28.7123) (10.0037, -28.6694) (10.0055, -28.6265) (10.0072, -28.5837) (10.0087, -28.541) (10.01, -28.4982) (10.0112, -28.4555) (10.0122, -28.4128) (10.0131, -28.3702) (10.0137, -28.3276) (10.0142, -28.285) (10.0145, -28.2425) (10.0146, -28.2) (10.0146, -28.1576) (10.0144, -28.1152) (10.0139, -28.0728) (10.0133, -28.0305) (10.0126, -27.9882) (10.0116, -27.946) (10.0104, -27.9038) (10.0091, -27.8617) (10.0075, -27.8196) (10.0057, -27.7775) (10.0038, -27.7355) (10.0016, -27.6936) (9.9993, -27.6517) (9.9967, -27.6099) (9.994, -27.5681) (9.991, -27.5264) (9.9878, -27.4847) (9.9843, -27.4431) (9.9807, -27.4015) (9.9768, -27.3601) (9.9727, -27.3186) (9.9683, -27.2773) (9.9638, -27.236) (9.9589, -27.1948) (9.9539, -27.1536) (9.9493, -27.1184) (9.9456, -27.0914) (9.943, -27.0727) (9.9415, -27.0622) (9.9412, -27.0598) knots -1 -1 -1 -1 -1 -1 -0.985714 -0.971429 -0.957143 -0.942857 -0.928571 -0.914286 -0.9 -0.885714 -0.871429 -0.857143 -0.842857 -0.828571 -0.814286 -0.8 -0.785714 -0.771429 -0.757143 -0.742857 -0.728571 -0.714286 -0.7 -0.685714 -0.671429 -0.657143 -0.642857 -0.628571 -0.614286 -0.6 -0.585714 -0.571429 -0.557143 -0.542857 -0.528571 -0.514286 -0.5 -0.485714 -0.471429 -0.457143 -0.442857 -0.428571 -0.414286 -0.4 -0.385714 -0.371429 -0.357143 -0.342857 -0.328571 -0.314286 -0.3 -0.285714 -0.271429 -0.257143 -0.242857 -0.228571 -0.224488 -0.224488 -0.224488 -0.224488 -0.224488 -0.224488
  spline S95 degree 3 poles (10.0054, -26.952) (9.9932, -26.9565) (9.982, -26.9634) (9.9628, -26.981) (9.9551, -26.9916) (9.9455, -27.0122) (9.9427, -27.0215) (9.9398, -27.0406) (9.9398, -27.0503) (9.9412, -27.0598) knots 0 0 0 0 0.003906 0.003906 0.007813 0.007813 0.010709 0.010709 0.013605 0.013605 0.013605 0.013605
  arc A78 (10.0054, -26.952) -> (10.599, -26.7241) centre (0, 0) ccw
  spline S96 degree 3 poles (10.7188, -26.7613) (10.7116, -26.7505) (10.7023, -26.7412) (10.6806, -26.7267) (10.6685, -26.7217) (10.6463, -26.7172) (10.6366, -26.7166) (10.6174, -26.7183) (10.6079, -26.7206) (10.599, -26.7241) knots 0 0 0 0 0.003906 0.003906 0.007813 0.007813 0.010709 0.010709 0.013605 0.013605 0.013605 0.013605
  spline S97 degree 5 poles (10.7188, -26.7613) (10.7202, -26.7633) (10.7261, -26.7721) (10.7367, -26.7878) (10.752, -26.8103) (10.7721, -26.8395) (10.7959, -26.8735) (10.8199, -26.9073) (10.8441, -26.9411) (10.8686, -26.9747) (10.8932, -27.0083) (10.9181, -27.0417) (10.9432, -27.075) (10.9685, -27.1082) (10.994, -27.1413) (11.0197, -27.1743) (11.0456, -27.2073) (11.0717, -27.2401) (11.098, -27.2728) (11.1244, -27.3054) (11.1511, -27.3379) (11.1779, -27.3703) (11.2049, -27.4026) (11.2321, -27.4348) (11.2595, -27.467) (11.287, -27.499) (11.3147, -27.5309) (11.3426, -27.5628) (11.3706, -27.5946) (11.3988, -27.6262) (11.4272, -27.6578) (11.4557, -27.6893) (11.4844, -27.7207) (11.5132, -27.752) (11.5422, -27.7832) (11.5714, -27.8143) (11.6007, -27.8454) (11.6301, -27.8763) (11.6597, -27.9072) (11.6895, -27.938) (11.7194, -27.9687) (11.7494, -27.9993) (11.7796, -28.0298) (11.8099, -28.0602) (11.8404, -28.0906) (11.871, -28.1208) (11.9018, -28.151) (11.9326, -28.1811) (11.9637, -28.2111) (11.9948, -28.241) (12.0261, -28.2709) (12.0576, -28.3006) (12.0891, -28.3303) (12.1208, -28.3599) (12.1527, -28.3894) (12.1846, -28.4188) (12.2103, -28.4423) (12.2296, -28.4599) (12.2425, -28.4716) (12.249, -28.4774) knots 0.224488 0.224488 0.224488 0.224488 0.224488 0.224488 0.228571 0.242857 0.257143 0.271429 0.285714 0.3 0.314286 0.328571 0.342857 0.357143 0.371429 0.385714 0.4 0.414286 0.428571 0.442857 0.457143 0.471429 0.485714 0.5 0.514286 0.528571 0.542857 0.557143 0.571429 0.585714 0.6 0.614286 0.628571 0.642857 0.657143 0.671429 0.685714 0.7 0.714286 0.728571 0.742857 0.757143 0.771429 0.785714 0.8 0.814286 0.828571 0.842857 0.857143 0.871429 0.885714 0.9 0.914286 0.928571 0.942857 0.957143 0.971429 0.985714 1 1 1 1 1 1
  arc A79 (12.249, -28.4774) -> (12.9667, -28.1579) centre (0, 0) ccw
  spline S98 degree 5 poles (12.9667, -28.1579) (12.9667, -28.1492) (12.9666, -28.1317) (12.9665, -28.1056) (12.9662, -28.0708) (12.9657, -28.0274) (12.9651, -27.984) (12.9643, -27.9407) (12.9634, -27.8973) (12.9623, -27.8541) (12.9611, -27.8108) (12.9597, -27.7677) (12.9581, -27.7245) (12.9565, -27.6814) (12.9546, -27.6384) (12.9526, -27.5954) (12.9504, -27.5524) (12.9481, -27.5095) (12.9456, -27.4667) (12.943, -27.4239) (12.9402, -27.3811) (12.9372, -27.3384) (12.9341, -27.2958) (12.9308, -27.2532) (12.9273, -27.2106) (12.9237, -27.1681) (12.9199, -27.1257) (12.9159, -27.0833) (12.9118, -27.041) (12.9075, -26.9987) (12.903, -26.9565) (12.8983, -26.9144) (12.8935, -26.8723) (12.8885, -26.8303) (12.8833, -26.7883) (12.8779, -26.7464) (12.8723, -26.7046) (12.8666, -26.6628) (12.8606, -26.6211) (12.8545, -26.5795) (12.8482, -26.5379) (12.8416, -26.4964) (12.8349, -26.455) (12.828, -26.4137) (12.8209, -26.3724) (12.8135, -26.3312) (12.806, -26.2901) (12.7982, -26.2491) (12.7902, -26.2082) (12.7821, -26.1673) (12.7736, -26.1265) (12.765, -26.0859) (12.7561, -26.0453) (12.747, -26.0048) (12.7377, -25.9644) (12.7294, -25.9299) (12.723, -25.9034) (12.7184, -25.8851) (12.7158, -25.8748) (12.7152, -25.8725) knots -1 -1 -1 -1 -1 -1 -0.985714 -0.971429 -0.957143 -0.942857 -0.928571 -0.914286 -0.9 -0.885714 -0.871429 -0.857143 -0.842857 -0.828571 -0.814286 -0.8 -0.785714 -0.771429 -0.757143 -0.742857 -0.728571 -0.714286 -0.7 -0.685714 -0.671429 -0.657143 -0.642857 -0.628571 -0.614286 -0.6 -0.585714 -0.571429 -0.557143 -0.542857 -0.528571 -0.514286 -0.5 -0.485714 -0.471429 -0.457143 -0.442857 -0.428571 -0.414286 -0.4 -0.385714 -0.371429 -0.357143 -0.342857 -0.328571 -0.314286 -0.3 -0.285714 -0.271429 -0.257143 -0.242857 -0.228571 -0.224488 -0.224488 -0.224488 -0.224488 -0.224488 -0.224488
  spline S99 degree 3 poles (12.7678, -25.7585) (12.7561, -25.7643) (12.7457, -25.7723) (12.7285, -25.7918) (12.7219, -25.8032) (12.7145, -25.8246) (12.7127, -25.8342) (12.7119, -25.8535) (12.7129, -25.8631) (12.7152, -25.8725) knots 0 0 0 0 0.003906 0.003906 0.007813 0.007813 0.010709 0.010709 0.013605 0.013605 0.013605 0.013605
  arc A80 (12.7678, -25.7585) -> (13.3343, -25.4698) centre (0, 0) ccw
  spline S100 degree 3 poles (13.4574, -25.4943) (13.4491, -25.4843) (13.4389, -25.476) (13.4158, -25.4639) (13.4032, -25.4601) (13.3807, -25.458) (13.371, -25.4584) (13.352, -25.4621) (13.3429, -25.4654) (13.3343, -25.4698) knots 0 0 0 0 0.003906 0.003906 0.007813 0.007813 0.010709 0.010709 0.013605 0.013605 0.013605 0.013605
  spline S101 degree 5 poles (13.4574, -25.4943) (13.459, -25.4961) (13.4658, -25.5043) (13.4779, -25.5187) (13.4955, -25.5395) (13.5186, -25.5665) (13.5458, -25.5978) (13.5732, -25.6289) (13.6008, -25.66) (13.6287, -25.6909) (13.6567, -25.7217) (13.6849, -25.7523) (13.7134, -25.7828) (13.742, -25.8132) (13.7708, -25.8435) (13.7998, -25.8736) (13.829, -25.9036) (13.8584, -25.9335) (13.8879, -25.9633) (13.9177, -25.993) (13.9476, -26.0225) (13.9776, -26.0519) (14.0079, -26.0813) (14.0383, -26.1105) (14.0689, -26.1396) (14.0996, -26.1685) (14.1305, -26.1974) (14.1615, -26.2262) (14.1927, -26.2548) (14.2241, -26.2834) (14.2556, -26.3118) (14.2873, -26.3401) (14.3191, -26.3684) (14.351, -26.3965) (14.3831, -26.4245) (14.4154, -26.4524) (14.4477, -26.4802) (14.4803, -26.5079) (14.5129, -26.5355) (14.5457, -26.563) (14.5787, -26.5904) (14.6118, -26.6177) (14.645, -26.6449) (14.6783, -26.672) (14.7118, -26.699) (14.7454, -26.7259) (14.7791, -26.7527) (14.813, -26.7794) (14.847, -26.806) (14.8811, -26.8325) (14.9154, -26.8589) (14.9497, -26.8852) (14.9842, -26.9115) (15.0188, -26.9376) (15.0536, -26.9636) (15.0884, -26.9895) (15.1164, -27.0102) (15.1375, -27.0256) (15.1515, -27.0359) (15.1586, -27.041) knots 0.224488 0.224488 0.224488 0.224488 0.224488 0.224488 0.228571 0.242857 0.257143 0.271429 0.285714 0.3 0.314286 0.328571 0.342857 0.357143 0.371429 0.385714 0.4 0.414286 0.428571 0.442857 0.457143 0.471429 0.485714 0.5 0.514286 0.528571 0.542857 0.557143 0.571429 0.585714 0.6 0.614286 0.628571 0.642857 0.657143 0.671429 0.685714 0.7 0.714286 0.728571 0.742857 0.757143 0.771429 0.785714 0.8 0.814286 0.828571 0.842857 0.857143 0.871429 0.885714 0.9 0.914286 0.928571 0.942857 0.957143 0.971429 0.985714 1 1 1 1 1 1
  arc A81 (15.1586, -27.041) -> (15.8389, -26.6482) centre (0, 0) ccw
  spline S102 degree 5 poles (15.8389, -26.6482) (15.838, -26.6396) (15.8361, -26.6223) (15.8333, -26.5963) (15.8294, -26.5617) (15.8244, -26.5186) (15.8192, -26.4755) (15.8139, -26.4325) (15.8084, -26.3895) (15.8028, -26.3466) (15.7971, -26.3037) (15.7912, -26.2609) (15.7852, -26.2181) (15.779, -26.1755) (15.7726, -26.1329) (15.7661, -26.0903) (15.7595, -26.0478) (15.7527, -26.0054) (15.7458, -25.963) (15.7387, -25.9207) (15.7314, -25.8785) (15.724, -25.8363) (15.7164, -25.7942) (15.7087, -25.7522) (15.7008, -25.7103) (15.6927, -25.6684) (15.6845, -25.6266) (15.6762, -25.5849) (15.6676, -25.5432) (15.6589, -25.5016) (15.65, -25.4601) (15.641, -25.4187) (15.6318, -25.3773) (15.6224, -25.3361) (15.6128, -25.2949) (15.6031, -25.2538) (15.5932, -25.2128) (15.5831, -25.1718) (15.5728, -25.131) (15.5624, -25.0902) (15.5517, -25.0495) (15.5409, -25.009) (15.5299, -24.9685) (15.5187, -24.9281) (15.5073, -24.8878) (15.4957, -24.8476) (15.4839, -24.8075) (15.4719, -24.7675) (15.4597, -24.7276) (15.4473, -24.6879) (15.4346, -24.6482) (15.4218, -24.6087) (15.4087, -24.5692) (15.3954, -24.5299) (15.3819, -24.4907) (15.3701, -24.4572) (15.3609, -24.4316) (15.3545, -24.4138) (15.3508, -24.4039) (15.35, -24.4016) knots -1 -1 -1 -1 -1 -1 -0.985714 -0.971429 -0.957143 -0.942857 -0.928571 -0.914286 -0.9 -0.885714 -0.871429 -0.857143 -0.842857 -0.828571 -0.814286 -0.8 -0.785714 -0.771429 -0.757143 -0.742857 -0.728571 -0.714286 -0.7 -0.685714 -0.671429 -0.657143 -0.642857 -0.628571 -0.614286 -0.6 -0.585714 -0.571429 -0.557143 -0.542857 -0.528571 -0.514286 -0.5 -0.485714 -0.471429 -0.457143 -0.442857 -0.428571 -0.414286 -0.4 -0.385714 -0.371429 -0.357143 -0.342857 -0.328571 -0.314286 -0.3 -0.285714 -0.271429 -0.257143 -0.242857 -0.228571 -0.224488 -0.224488 -0.224488 -0.224488 -0.224488 -0.224488
  spline S103 degree 3 poles (15.3904, -24.2828) (15.3794, -24.2898) (15.3698, -24.2988) (15.3548, -24.3201) (15.3494, -24.332) (15.3443, -24.3541) (15.3435, -24.3638) (15.3447, -24.3831) (15.3467, -24.3926) (15.35, -24.4016) knots 0 0 0 0 0.003906 0.003906 0.007813 0.007813 0.010709 0.010709 0.013605 0.013605 0.013605 0.013605
  arc A82 (15.3904, -24.2828) -> (15.9236, -23.9365) centre (0, 0) ccw
  spline S104 degree 3 poles (16.0486, -23.948) (16.0393, -23.9389) (16.0282, -23.9317) (16.004, -23.9221) (15.9911, -23.9196) (15.9685, -23.9198) (15.9589, -23.9213) (15.9404, -23.927) (15.9316, -23.9311) (15.9236, -23.9365) knots 0 0 0 0 0.003906 0.003906 0.007813 0.007813 0.010709 0.010709 0.013605 0.013605 0.013605 0.013605
  spline S105 degree 5 poles (16.0486, -23.948) (16.0503, -23.9496) (16.0579, -23.957) (16.0715, -23.9701) (16.0912, -23.9889) (16.117, -24.0133) (16.1473, -24.0416) (16.1778, -24.0698) (16.2085, -24.0977) (16.2394, -24.1256) (16.2705, -24.1532) (16.3018, -24.1808) (16.3333, -24.2081) (16.3649, -24.2354) (16.3967, -24.2625) (16.4288, -24.2894) (16.4609, -24.3162) (16.4933, -24.3429) (16.5258, -24.3694) (16.5584, -24.3958) (16.5913, -24.422) (16.6242, -24.4482) (16.6574, -24.4742) (16.6907, -24.5) (16.7241, -24.5258) (16.7577, -24.5514) (16.7915, -24.5769) (16.8253, -24.6022) (16.8594, -24.6275) (16.8935, -24.6526) (16.9278, -24.6776) (16.9623, -24.7024) (16.9969, -24.7272) (17.0316, -24.7518) (17.0664, -24.7763) (17.1014, -24.8007) (17.1365, -24.825) (17.1718, -24.8491) (17.2072, -24.8732) (17.2426, -24.8971) (17.2783, -24.9209) (17.314, -24.9446) (17.3499, -24.9682) (17.3859, -24.9916) (17.422, -25.015) (17.4582, -25.0382) (17.4946, -25.0613) (17.5311, -25.0843) (17.5677, -25.1072) (17.6044, -25.13) (17.6412, -25.1527) (17.6781, -25.1753) (17.7152, -25.1978) (17.7523, -25.2201) (17.7896, -25.2424) (17.827, -25.2645) (17.857, -25.2821) (17.8795, -25.2953) (17.8946, -25.304) (17.9021, -25.3084) knots 0.224488 0.224488 0.224488 0.224488 0.224488 0.224488 0.228571 0.242857 0.257143 0.271429 0.285714 0.3 0.314286 0.328571 0.342857 0.357143 0.371429 0.385714 0.4 0.414286 0.428571 0.442857 0.457143 0.471429 0.485714 0.5 0.514286 0.528571 0.542857 0.557143 0.571429 0.585714 0.6 0.614286 0.628571 0.642857 0.657143 0.671429 0.685714 0.7 0.714286 0.728571 0.742857 0.757143 0.771429 0.785714 0.8 0.814286 0.828571 0.842857 0.857143 0.871429 0.885714 0.9 0.914286 0.928571 0.942857 0.957143 0.971429 0.985714 1 1 1 1 1 1
  arc A83 (17.9021, -25.3084) -> (18.5377, -24.8466) centre (0, 0) ccw
  spline S106 degree 5 poles (18.5377, -24.8466) (18.5358, -24.8381) (18.5322, -24.8211) (18.5266, -24.7956) (18.5191, -24.7616) (18.5096, -24.7192) (18.5, -24.6769) (18.4902, -24.6347) (18.4803, -24.5925) (18.4702, -24.5504) (18.46, -24.5083) (18.4497, -24.4664) (18.4392, -24.4245) (18.4286, -24.3827) (18.4179, -24.341) (18.407, -24.2994) (18.3959, -24.2578) (18.3847, -24.2163) (18.3734, -24.1749) (18.3619, -24.1336) (18.3503, -24.0924) (18.3385, -24.0512) (18.3265, -24.0101) (18.3145, -23.9692) (18.3022, -23.9283) (18.2899, -23.8874) (18.2773, -23.8467) (18.2646, -23.8061) (18.2518, -23.7656) (18.2388, -23.7251) (18.2256, -23.6848) (18.2123, -23.6445) (18.1988, -23.6044) (18.1851, -23.5643) (18.1713, -23.5243) (18.1574, -23.4845) (18.1432, -23.4447) (18.1289, -23.405) (18.1144, -23.3655) (18.0998, -23.3261) (18.0849, -23.2867) (18.0699, -23.2475) (18.0547, -23.2084) (18.0394, -23.1694) (18.0238, -23.1305) (18.0081, -23.0917) (17.9922, -23.0531) (17.976, -23.0146) (17.9597, -22.9762) (17.9432, -22.938) (17.9265, -22.8998) (17.9096, -22.8618) (17.8925, -22.824) (17.8752, -22.7863) (17.8576, -22.7487) (17.8424, -22.7166) (17.8306, -22.6921) (17.8223, -22.6751) (17.8176, -22.6656) (17.8166, -22.6635) knots -1 -1 -1 -1 -1 -1 -0.985714 -0.971429 -0.957143 -0.942857 -0.928571 -0.914286 -0.9 -0.885714 -0.871429 -0.857143 -0.842857 -0.828571 -0.814286 -0.8 -0.785714 -0.771429 -0.757143 -0.742857 -0.728571 -0.714286 -0.7 -0.685714 -0.671429 -0.657143 -0.642857 -0.628571 -0.614286 -0.6 -0.585714 -0.571429 -0.557143 -0.542857 -0.528571 -0.514286 -0.5 -0.485714 -0.471429 -0.457143 -0.442857 -0.428571 -0.414286 -0.4 -0.385714 -0.371429 -0.357143 -0.342857 -0.328571 -0.314286 -0.3 -0.285714 -0.271429 -0.257143 -0.242857 -0.228571 -0.224488 -0.224488 -0.224488 -0.224488 -0.224488 -0.224488
  spline S107 degree 3 poles (17.8443, -22.541) (17.8341, -22.5491) (17.8255, -22.5591) (17.8128, -22.5818) (17.8087, -22.5943) (17.8059, -22.6168) (17.8061, -22.6265) (17.8093, -22.6455) (17.8123, -22.6548) (17.8166, -22.6635) knots 0 0 0 0 0.003906 0.003906 0.007813 0.007813 0.010709 0.010709 0.013605 0.013605 0.013605 0.013605
  arc A84 (17.8443, -22.541) -> (18.3384, -22.1409) centre (0, 0) ccw
  spline S108 degree 3 poles (18.4639, -22.1392) (18.4537, -22.1312) (18.442, -22.1252) (18.4169, -22.1181) (18.4038, -22.1171) (18.3813, -22.1196) (18.3719, -22.1221) (18.3541, -22.1297) (18.3458, -22.1347) (18.3384, -22.1409) knots 0 0 0 0 0.003906 0.003906 0.007813 0.007813 0.010709 0.010709 0.013605 0.013605 0.013605 0.013605
  spline S109 degree 5 poles (18.4639, -22.1392) (18.4658, -22.1407) (18.4742, -22.1473) (18.4891, -22.1589) (18.5106, -22.1755) (18.5388, -22.1971) (18.5719, -22.2221) (18.6052, -22.2469) (18.6386, -22.2715) (18.6723, -22.2959) (18.7061, -22.3202) (18.7401, -22.3443) (18.7742, -22.3682) (18.8086, -22.392) (18.843, -22.4156) (18.8777, -22.4391) (18.9125, -22.4624) (18.9474, -22.4855) (18.9825, -22.5085) (19.0178, -22.5313) (19.0532, -22.554) (19.0887, -22.5765) (19.1244, -22.5989) (19.1602, -22.6212) (19.1961, -22.6433) (19.2322, -22.6652) (19.2684, -22.687) (19.3048, -22.7087) (19.3413, -22.7303) (19.3779, -22.7517) (19.4146, -22.7729) (19.4515, -22.7941) (19.4885, -22.8151) (19.5256, -22.8359) (19.5628, -22.8567) (19.6001, -22.8773) (19.6376, -22.8977) (19.6752, -22.9181) (19.7128, -22.9383) (19.7506, -22.9583) (19.7886, -22.9783) (19.8266, -22.9981) (19.8647, -23.0178) (19.903, -23.0374) (19.9413, -23.0568) (19.9798, -23.0762) (20.0184, -23.0954) (20.0571, -23.1144) (20.0958, -23.1334) (20.1347, -23.1522) (20.1737, -23.1709) (20.2128, -23.1895) (20.252, -23.208) (20.2913, -23.2263) (20.3307, -23.2446) (20.3702, -23.2627) (20.4018, -23.2771) (20.4256, -23.2878) (20.4415, -23.2949) (20.4495, -23.2985) knots 0.224488 0.224488 0.224488 0.224488 0.224488 0.224488 0.228571 0.242857 0.257143 0.271429 0.285714 0.3 0.314286 0.328571 0.342857 0.357143 0.371429 0.385714 0.4 0.414286 0.428571 0.442857 0.457143 0.471429 0.485714 0.5 0.514286 0.528571 0.542857 0.557143 0.571429 0.585714 0.6 0.614286 0.628571 0.642857 0.657143 0.671429 0.685714 0.7 0.714286 0.728571 0.742857 0.757143 0.771429 0.785714 0.8 0.814286 0.828571 0.842857 0.857143 0.871429 0.885714 0.9 0.914286 0.928571 0.942857 0.957143 0.971429 0.985714 1 1 1 1 1 1
  arc A85 (20.4495, -23.2985) -> (21.0333, -22.7728) centre (0, 0) ccw
  spline S110 degree 5 poles (21.0333, -22.7728) (21.0306, -22.7645) (21.0252, -22.748) (21.017, -22.7232) (21.006, -22.6902) (20.9921, -22.649) (20.9781, -22.6079) (20.9639, -22.5669) (20.9497, -22.526) (20.9353, -22.4852) (20.9207, -22.4445) (20.9061, -22.4038) (20.8913, -22.3633) (20.8763, -22.3228) (20.8613, -22.2825) (20.8461, -22.2422) (20.8308, -22.202) (20.8153, -22.1619) (20.7997, -22.1219) (20.7839, -22.082) (20.7681, -22.0423) (20.7521, -22.0026) (20.7359, -21.963) (20.7196, -21.9235) (20.7032, -21.8841) (20.6866, -21.8448) (20.6699, -21.8056) (20.653, -21.7665) (20.636, -21.7275) (20.6188, -21.6887) (20.6015, -21.6499) (20.584, -21.6113) (20.5664, -21.5728) (20.5487, -21.5343) (20.5308, -21.496) (20.5127, -21.4579) (20.4945, -21.4198) (20.4761, -21.3818) (20.4575, -21.344) (20.4388, -21.3063) (20.42, -21.2688) (20.401, -21.2313) (20.3818, -21.194) (20.3624, -21.1568) (20.3429, -21.1198) (20.3232, -21.0829) (20.3033, -21.0461) (20.2833, -21.0095) (20.263, -20.973) (20.2426, -20.9367) (20.222, -20.9006) (20.2012, -20.8645) (20.1802, -20.8287) (20.159, -20.793) (20.1377, -20.7575) (20.1192, -20.7271) (20.1049, -20.704) (20.0949, -20.688) (20.0892, -20.679) (20.0879, -20.677) knots -1 -1 -1 -1 -1 -1 -0.985714 -0.971429 -0.957143 -0.942857 -0.928571 -0.914286 -0.9 -0.885714 -0.871429 -0.857143 -0.842857 -0.828571 -0.814286 -0.8 -0.785714 -0.771429 -0.757143 -0.742857 -0.728571 -0.714286 -0.7 -0.685714 -0.671429 -0.657143 -0.642857 -0.628571 -0.614286 -0.6 -0.585714 -0.571429 -0.557143 -0.542857 -0.528571 -0.514286 -0.5 -0.485714 -0.471429 -0.457143 -0.442857 -0.428571 -0.414286 -0.4 -0.385714 -0.371429 -0.357143 -0.342857 -0.328571 -0.314286 -0.3 -0.285714 -0.271429 -0.257143 -0.242857 -0.228571 -0.224488 -0.224488 -0.224488 -0.224488 -0.224488 -0.224488
  spline S111 degree 3 poles (20.1027, -20.5523) (20.0934, -20.5614) (20.086, -20.5722) (20.0757, -20.5962) (20.0729, -20.609) (20.0725, -20.6317) (20.0737, -20.6413) (20.0789, -20.6599) (20.0828, -20.6688) (20.0879, -20.677) knots 0 0 0 0 0.003906 0.003906 0.007813 0.007813 0.010709 0.010709 0.013605 0.013605 0.013605 0.013605
  arc A86 (20.1027, -20.5523) -> (20.5523, -20.1027) centre (0, 0) ccw